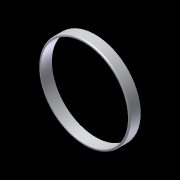
# Autodesk Inventor part: Wheel_Rim
Saved by Autodesk Inventor 2011 SP1 (Build 150282100, 282)
## iProperties
Created: 2013-01-14
Part Number: Wheel_Rim
Material: Rubber
Document SubType Name: Modeling
Designer: 939551
Mass: 63.8453 g
Surface Area: 358.382 cm^2
Volume: 68.6509 cm^3
Density: 0.93 g/cm^3
Author: 939551
Autodesk Inventor part; units mm, degrees
ref_plane "YZ Plane" through (0, 0, 0) normal (1, 0, 0) x (0, 1, 0)
ref_plane "XZ Plane" through (0, 0, 0) normal (0, 1, 0) x (-1, 0, 0)
ref_plane "XY Plane" through (0, 0, 0) normal (0, 0, 1) x (1, 0, 0)
sketch "Sketch1" plane through (0, 0, 0) normal (0, 0, 1) x (1, 0, 0)
  circle A0 centre (0, 0) radius 101.6
  circle A1 centre (0, 0) radius 97.155
  dimension "d0" = 203.2
  dimension "d1" = 194.31
  constraints: 2 centre point, 2 coincident
  measures "d0" diameter of A0
  measures "d1" diameter of A1
extrude "Extrusion1" add sketch "Sketch1" along normal blind 25.4
fillet "Fillet1" radius 2.6035 2 edges at (-101.6, 0, 25.4) (-101.6, 0, 0)
body "Solid1"
